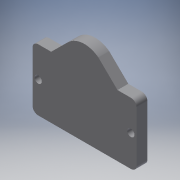
# Autodesk Inventor part: headplateLP_protector
Saved by Autodesk Inventor 2016 (Build 200138000, 138)
## iProperties
Created: 2009-03-31
Part Number: headplateLP_protector
Document SubType Name: Modeling
Designer: Daniel
Material: Generic
Density: 1 g/cm^3
Appearance: Default
Author: Daniel
Autodesk Inventor part; units mm, degrees
ref_plane "YZ Plane" through (0, 0, 0) normal (1, 0, 0) x (0, 1, 0)
ref_plane "XZ Plane" through (0, 0, 0) normal (0, 1, 0) x (-1, 0, 0)
ref_plane "XY Plane" through (0, 0, 0) normal (0, 0, 1) x (1, 0, 0)
sketch "Block1" plane through (0, 0, 0) normal (0, 0, 1) x (1, 0, 0)
  line L0 (-17.5911, -8.406) -> (-17.5911, -2.6569)
  arc A0 (-15.6308, 0.6431) -> (-17.4939, -2.2845) centre (9.5285, -17.4245) ccw
  arc A1 (-17.4939, -2.2845) -> (-17.5911, -2.6569) centre (-16.8291, -2.6569) ccw
  line L1 (-13.0521, -3.6322) -> (-2.9855, -3.6322)
  line L2 (-2.9855, -3.6322) -> (-2.9855, -10.0136)
  line L3 (-2.9855, -10.0136) -> (-13.0521, -10.0136)
  line L4 (-13.0521, -10.0136) -> (-13.0521, -3.6322)
  ellipse E0 centre (-8.0188, -3.6322) end of major axis (-8.0188, -7.4704) minor radius 2.9685
  point P0 (-13.9703, -5.5207)
  point P1 (-17.5911, -2.4593)
  dimension "d111" = 0.762
  measures "d111" radius of A1
sketch "Block2" plane through (0, 0, 0) normal (0, 0, 1) x (1, 0, 0)
  line L0 (-7.8958, -2.4967) -> (-7.8958, -8.4058)
  line L1 (-8.6339, -9.168) -> (-16.8291, -9.168)
  ellipse E0 centre (-12.6564, -2.1178) end of major axis (-12.6564, -6.4967) minor radius 3.853 (-9.6585, 0.6329) -> (-15.6415, 0.6509) ccw
  arc A0 (-7.8958, -2.4967) -> (-9.6091, 0.6391) centre (-35.8892, -15.7554) ccw
  line L2 (-17.6018, -8.3981) -> (-17.6018, -2.6491)
  arc A1 (-15.6415, 0.6509) -> (-17.5045, -2.2766) centre (9.5178, -17.4167) ccw
  arc A2 (-17.5045, -2.2766) -> (-17.6018, -2.6491) centre (-16.8398, -2.6491) ccw
  line L3 (-13.0627, -3.6243) -> (-2.9962, -3.6243)
  line L4 (-2.9962, -3.6243) -> (-2.9962, -10.0058)
  line L5 (-2.9962, -10.0058) -> (-13.0627, -10.0058)
  line L6 (-13.0627, -10.0058) -> (-13.0627, -3.6243)
  ellipse E1 centre (-8.0295, -3.6243) end of major axis (-8.0295, -7.4625) minor radius 2.9685
  point P0 (-12.2397, -5.1213)
sketch "Block3" plane through (0, 0, 0) normal (0, 0, 1) x (1, 0, 0)
  arc A0 (-17.5911, -8.406) -> (-16.8291, -9.168) centre (-16.8291, -8.406) ccw
  arc A1 (-8.6339, -9.168) -> (-7.8719, -8.406) centre (-8.6339, -8.406) ccw
  line L0 (-7.8958, -2.4967) -> (-7.8958, -8.4058)
  line L1 (-8.6339, -9.168) -> (-16.8291, -9.168)
  ellipse E0 centre (-12.6564, -2.1178) end of major axis (-12.6564, -6.4967) minor radius 3.853 (-9.6585, 0.6329) -> (-15.6415, 0.6509) ccw
  arc A2 (-7.8958, -2.4967) -> (-9.6091, 0.6391) centre (-35.8892, -15.7554) ccw
  line L2 (-17.6018, -8.3981) -> (-17.6018, -2.6491)
  arc A3 (-15.6415, 0.6509) -> (-17.5045, -2.2766) centre (9.5178, -17.4167) ccw
  arc A4 (-17.5045, -2.2766) -> (-17.6018, -2.6491) centre (-16.8398, -2.6491) ccw
  line L3 (-13.0627, -3.6243) -> (-2.9962, -3.6243)
  line L4 (-2.9962, -3.6243) -> (-2.9962, -10.0058)
  line L5 (-2.9962, -10.0058) -> (-13.0627, -10.0058)
  line L6 (-13.0627, -10.0058) -> (-13.0627, -3.6243)
  ellipse E1 centre (-8.0295, -3.6243) end of major axis (-8.0295, -7.4625) minor radius 2.9685
  point P0 (-12.6868, -8.3844)
  dimension "d110" = 0.762
  measures "d110" radius of A0
sketch "Block4" plane through (0, 0, 0) normal (0, 0, 1) x (1, 0, 0)
  arc A0 (-17.5911, -8.406) -> (-16.8291, -9.168) centre (-16.8291, -8.406) ccw
  arc A1 (-8.6339, -9.168) -> (-7.8719, -8.406) centre (-8.6339, -8.406) ccw
  line L0 (-7.8958, -2.4967) -> (-7.8958, -8.4058)
  line L1 (-8.6339, -9.168) -> (-16.8291, -9.168)
  ellipse E0 centre (-12.6564, -2.1178) end of major axis (-12.6564, -6.4967) minor radius 3.853 (-9.6585, 0.6329) -> (-15.6415, 0.6509) ccw
  arc A2 (-7.8958, -2.4967) -> (-9.6091, 0.6391) centre (-35.8892, -15.7554) ccw
  line L2 (-17.6018, -8.3981) -> (-17.6018, -2.6491)
  arc A3 (-15.6415, 0.6509) -> (-17.5045, -2.2766) centre (9.5178, -17.4167) ccw
  arc A4 (-17.5045, -2.2766) -> (-17.6018, -2.6491) centre (-16.8398, -2.6491) ccw
  line L3 (-13.0627, -3.6243) -> (-2.9962, -3.6243)
  line L4 (-2.9962, -3.6243) -> (-2.9962, -10.0058)
  line L5 (-2.9962, -10.0058) -> (-13.0627, -10.0058)
  line L6 (-13.0627, -10.0058) -> (-13.0627, -3.6243)
  ellipse E1 centre (-8.0295, -3.6243) end of major axis (-8.0295, -7.4625) minor radius 2.9685
  point P0 (-12.6868, -8.3844)
sketch "Block5" plane through (0, 0, 0) normal (0, 0, 1) x (1, 0, 0)
  ellipse E0 centre (-12.7876, -1.8459) end of major axis (-12.7876, -5.6516) minor radius 3.3457 (-10.6846, 1.114) -> (-14.8941, 1.1109) ccw
  arc A0 (-15.6984, 0.3796) -> (-14.8859, 1.1184) centre (-85.8065, 78.298) ccw
  arc A1 (-10.6894, 1.1184) -> (-9.8669, 0.3716) centre (60.1779, 78.3469) ccw
  point P0 (-12.7899, 8.9309)
sketch "Block6" plane through (0, 0, 0) normal (0, 0, 1) x (1, 0, 0)
  arc A0 (-10.9697, 1.4333) -> (-15.1792, 1.1122) centre (-12.8849, -1.2117) ccw
  line L0 (-15.1792, 1.1122) -> (-17.7718, -1.4473)
  line L1 (-10.8839, 1.361) -> (-8.0119, -1.4473)
  line L2 (-17.7718, -1.4473) -> (-8.0119, -1.4473)
  arc A1 (-10.8839, 1.361) -> (-10.9697, 1.4333) centre (-11.4166, 0.8161) ccw
  point P0 (-12.0633, -0.3449)
  point P1 (-10.9214, 1.3977)
  dimension "d153" = 0.762
  measures "d153" radius of A1
sketch "Sketch1" plane through (0, 0, 0) normal (0, 0, 1) x (1, 0, 0)
  line L0 (-19.9256, -1.4064) -> (-6.1106, -1.4064)
  line L1 (-6.1106, -1.4064) -> (-6.1106, -8.6156)
  line L2 (-6.1106, -8.6156) -> (-19.9256, -8.6156)
  line L3 (-19.9256, -8.6156) -> (-19.9256, -1.4064)
  constraints: 8 end point, 2 parallel, 1 horizontal, 1 perpendicular
extrude "Extrusion1" add sketch "Sketch1" along normal blind 1.524
sketch "Sketch13" plane through (0, 0, 1.524) normal (0, 0, 1) x (1, 0, 0)
  arc A0 (-10.8192, 2.023) -> (-15.0287, 1.7019) centre (-12.7344, -0.622) ccw
  line L0 (-15.0287, 1.7019) -> (-17.6213, -0.8576)
  line L1 (-10.7334, 1.9507) -> (-7.8614, -0.8576)
  line L2 (-17.6213, -0.8576) -> (-7.8614, -0.8576)
  arc A1 (-10.7334, 1.9507) -> (-10.8192, 2.023) centre (-11.2661, 1.4058) ccw
  point P0 (0, 0)
  point P1 (0, 0)
  point P2 (0, 0)
extrude "Extrusion8" add sketch "Sketch13" against normal blind 1.524
sketch "Sketch16" plane through (0, 0, 1.524) normal (0, 0, 1) x (1, 0, 0)
  line L0 (-19.2542, -0.6452) -> (-6.1548, -0.6452)
  line L1 (-5.3928, -1.4072) -> (-5.3928, -8.5513)
  line L2 (-6.1548, -9.3133) -> (-19.2542, -9.3133)
  line L3 (-20.0162, -8.5513) -> (-20.0162, -1.4072)
  arc A0 (-19.2542, -0.6452) -> (-20.0162, -1.4072) centre (-19.2542, -1.4072) ccw
  arc A1 (-20.0162, -8.5513) -> (-19.2542, -9.3133) centre (-19.2542, -8.5513) ccw
  arc A2 (-6.1548, -9.3133) -> (-5.3928, -8.5513) centre (-6.1548, -8.5513) ccw
  arc A3 (-5.3928, -1.4072) -> (-6.1548, -0.6452) centre (-6.1548, -1.4072) ccw
  point P0 (0, 0)
  dimension "d177" = 0.762
  dimension "d178" = 0.762
  dimension "d179" = 0.762
  dimension "d180" = 0.762
  constraints: 8 end point, 8 point on circle, 8 tangent, 4 centre point, 2 parallel, 1 horizontal, 1 perpendicular
  measures "d177" radius of A0
  measures "d178" radius of A1
  measures "d179" radius of A2
  measures "d180" radius of A3
extrude "Extrusion9" add sketch "Sketch16" against normal blind 1.524
hole "Hole9" at (-19.2355, -4.93, 1.524) direction (0, 0, -1) diameter 1.016 depth 1.524
hole "Hole10" at (-6.1975, -4.9172, 1.524) direction (0, 0, -1) diameter 1.016 depth 1.524
body "Solid1"
